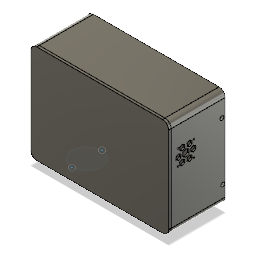
mouse_mock_MRI_box (Autodesk Fusion 360 design; units mm, degrees)
Autodesk Fusion 360 part; units mm, degrees
sketch "Sketch1" plane through (0, 0, 0) normal (0, 0, 1) x (1, 0, 0)
  line L0 (-140, 100) -> (140, 100)
  line L1 (140, 100) -> (140, -100)
  line L2 (140, -100) -> (-140, -100)
  line L3 (-140, -100) -> (-140, 100)
  line L4 (137, -97) -> (-137, -97)
  line L5 (-137, -97) -> (-137, 97)
  line L6 (-137, 97) -> (137, 97)
  line L7 (137, 97) -> (137, -97)
  dimension "d1" = 140
  dimension "d2" = 280
  dimension "d3" = 100
  dimension "d4" = 200
  dimension "d5" = 3
  constraint horizontal L0
  constraint vertical L1
  constraint horizontal L2
  constraint vertical L3
  measures "d1" distance of origin L3
  measures "d2" distance of L0.start L0.end
  measures "d3" distance of origin L0
  measures "d4" distance of L0.start L2.end
extrude "Extrude1" add sketch "Sketch1" along normal blind 10 contours L4 L5 L6 L7 makes body 1
extrude "Extrude2" add sketch "Sketch1" along normal blind 110 bodies 1
sketch "Sketch2" plane through (0, 0, 10) normal (0, 0, 1) x (1, 0, 0)
  line L0 (137, 97) -> (-137, 97)
  line L1 (-137, 97) -> (-137, -97)
  line L2 (-137, -97) -> (137, -97)
  line L3 (137, -97) -> (137, 97)
  line L4 (-30.5, 80) -> (-55.5, 80)
  line L5 (-55.5, 80) -> (-55.5, 10)
  line L6 (-55.5, 10) -> (-30.5, 10)
  line L7 (-30.5, 10) -> (-30.5, 80)
  line L8 (30.5, 80) -> (55.5, 80)
  line L9 (55.5, 80) -> (55.5, 10)
  line L10 (55.5, 10) -> (30.5, 10)
  line L11 (30.5, 10) -> (30.5, 80)
  line L12 (-9.5, -65) -> (9.5, -65)
  line L13 (9.5, -65) -> (9.5, -75.5)
  line L14 (9.5, -75.5) -> (-9.5, -75.5)
  line L15 (-9.5, -75.5) -> (-9.5, -65)
  circle A0 centre (-12.5, -70.25) radius 1.5
  circle A1 centre (12.5, -70.25) radius 1.5
  line L16 (-76.5, -65) -> (-95.5, -65)
  line L17 (-95.5, -65) -> (-95.5, -75.5)
  line L18 (-95.5, -75.5) -> (-76.5, -75.5)
  line L19 (-76.5, -75.5) -> (-76.5, -65)
  circle A2 centre (-73.5, -70.25) radius 1.5
  circle A3 centre (-98.5, -70.25) radius 1.5
  line L20 (0, 0) -> (0, -11.4681)
  circle A4 centre (98.5, -70.25) radius 1.5
  line L21 (95.5, -65) -> (95.5, -75.5)
  line L22 (95.5, -75.5) -> (76.5, -75.5)
  line L23 (76.5, -65) -> (95.5, -65)
  line L24 (76.5, -75.5) -> (76.5, -65)
  circle A5 centre (73.5, -70.25) radius 1.5
  line L25 (-116.5, 80) -> (-126.5, 80)
  line L26 (-126.5, 80) -> (-126.5, 10)
  line L27 (-126.5, 10) -> (-116.5, 10)
  line L28 (-116.5, 10) -> (-116.5, 80)
  line L29 (126.5, 80) -> (126.5, 10)
  line L30 (116.5, 80) -> (126.5, 80)
  line L31 (116.5, 10) -> (116.5, 80)
  line L32 (126.5, 10) -> (116.5, 10)
  line L33 (137, -97) -> (-137, -97)
  line L34 (-137, -97) -> (-137, -82.25)
  line L35 (-137, -82.25) -> (137, -82.25)
  line L36 (137, -82.25) -> (137, -97)
  line L37 (-116.5, -82.25) -> (-126.5, -82.25)
  line L38 (-126.5, -82.25) -> (-126.5, -72.25)
  line L39 (-126.5, -72.25) -> (-116.5, -72.25)
  line L40 (-116.5, -72.25) -> (-116.5, -82.25)
  line L41 (126.5, -82.25) -> (126.5, -72.25)
  line L42 (126.5, -72.25) -> (116.5, -72.25)
  line L43 (116.5, -72.25) -> (116.5, -82.25)
  line L44 (-30.5, -82.25) -> (-55.5, -82.25)
  line L45 (-55.5, -82.25) -> (-55.5, -72.25)
  line L46 (-55.5, -72.25) -> (-30.5, -72.25)
  line L47 (-30.5, -72.25) -> (-30.5, -82.25)
  line L48 (55.5, -82.25) -> (55.5, -72.25)
  line L49 (55.5, -72.25) -> (30.5, -72.25)
  line L50 (30.5, -72.25) -> (30.5, -82.25)
  dimension "d10" = 70
  dimension "d11" = 25
  dimension "d12" = 70
  dimension "d13" = 25
  dimension "d14" = 30.5
  dimension "d15" = 30.5
  dimension "d16" = 19
  dimension "d17" = 10.5
  dimension "d18" = 9.5
  dimension "d19" = 65
  dimension "d20" = 3
  dimension "d21" = 3
  dimension "d22" = 25
  dimension "d23" = 12.5
  dimension "d24" = 5.25
  dimension "d25" = 5.25
  dimension "d26" = 19
  dimension "d27" = 10.5
  dimension "d28" = 80
  dimension "d29" = 65
  dimension "d30" = 21
  dimension "d31" = 3
  dimension "d32" = 3
  dimension "d33" = 5.25
  dimension "d34" = 5.25
  dimension "d35" = 25
  dimension "d36" = 3
  dimension "d46" = 70
  dimension "d47" = 61
  dimension "d48" = 10
  dimension "d85" = 80
  dimension "d86" = 80
  dimension "d87" = 12
  dimension "d93" = 10
  dimension "d94" = 10
  constraint horizontal L4
  constraint vertical L5
  constraint horizontal L6
  constraint vertical L7
  constraint horizontal L8
  constraint vertical L9
  constraint horizontal L10
  constraint vertical L11
  constraint horizontal L12
  constraint vertical L13
  constraint horizontal L14
  constraint vertical L15
  constraint horizontal L16
  constraint vertical L17
  constraint horizontal L18
  constraint vertical L19
  constraint coincident L20.start origin
  constraint vertical L20
  constraint symmetric L16.start L20 L23.start
  constraint symmetric L16.end L20 L21.start
  constraint symmetric L17.end L20 L21.end
  constraint symmetric L18.end L20 L22.end
  constraint symmetric A2 L20 A5
  constraint symmetric A3 L20 A4
  constraint horizontal L25
  constraint vertical L26
  constraint horizontal L27
  constraint vertical L28
  constraint symmetric L20 L25.start L30.start
  constraint symmetric L20 L25.end L29.start
  constraint symmetric L20 L26.end L29.end
  constraint symmetric L20 L27.end L31.start
  constraint horizontal L33
  constraint vertical L34
  constraint horizontal L35
  constraint vertical L36
  constraint coincident L2 L3.start
  constraint coincident L1 L2.start
  constraint coincident L2.end L36
  constraint horizontal L37
  constraint vertical L38
  constraint horizontal L39
  constraint vertical L40
  constraint coincident L35 L37.start
  constraint symmetric L20 L37.start L43.end
  constraint symmetric L20 L37.end L41.start
  constraint symmetric L20 L38.end L41.end
  constraint symmetric L20 L39.end L42.end
  constraint horizontal L44
  constraint vertical L45
  constraint horizontal L46
  constraint vertical L47
  constraint coincident L35 L44.start
  constraint symmetric L20 L44.start L50.end
  constraint symmetric L20 L44.end L48.start
  constraint symmetric L20 L45.end L48.end
  constraint symmetric L20 L46.end L49.end
  measures "d10" distance of L4.start L6.end
  measures "d11" distance of L4.start L4.end
  measures "d12" distance of L8.start L10.end
  measures "d13" distance of L8.start L8.end
  measures "d14" distance of L20.start L7
  measures "d15" distance of L20.start L11
  measures "d16" distance of L12.start L12.end
  measures "d17" distance of L12.start L14.end
  measures "d18" distance of L20.start L15
  measures "d19" distance of L20.start L12
  measures "d20" diameter of A0
  measures "d21" diameter of A1
  measures "d22" distance of A0.centre A1.centre
  measures "d23" horizontal distance of L20.start A0.centre
  measures "d24" distance of L12 A0.centre
  measures "d25" distance of L12 A1.centre
  measures "d26" distance of L16.start L16.end
  measures "d27" distance of L16.start L18.end
  measures "d28" distance of L20.start L4
  measures "d29" distance of L20.start L16
  measures "d30" distance of L5 L19
  measures "d31" diameter of A2
  measures "d32" diameter of A3
  measures "d33" distance of L16 A2.centre
  measures "d34" distance of L16 A3.centre
  measures "d35" distance of A2.centre A3.centre
  measures "d36" distance of L17 A3.centre
  measures "d46" distance of L25.start L27.end
  measures "d47" distance of L5 L28
  measures "d48" distance of L25.start L25.end
  measures "d85" distance of L20.start L8
  measures "d86" distance of L20.start L25
  measures "d87" distance of A2.centre L35
  measures "d93" distance of L37.start L39.end
  measures "d94" distance of L44.start L46.end
extrude "Extrude3" add sketch "Sketch2" along normal blind 20 contours L4 L5 L6 L7 | L8 L9 L10 L11 | L25 L26 L27 L28 | L29 L30 L31 L32 bodies 1
extrude "Extrude4" cut sketch "Sketch2" against normal blind 9 contours L12 L13 L14 L15 | A0 | A1 | L16 L17 L18 L19 | A2 | A3 | A4 | L21 L22 L23 L24 | A5 bodies 1
sketch "Sketch3" plane through (140, 0, 0) normal (1, 0, 0) x (0, 0, -1)
  line L0 (0, -100) -> (0, 100)
  line L1 (0, 100) -> (-110, 100)
  line L2 (-110, 100) -> (-110, -100)
  line L3 (-110, -100) -> (0, -100)
  circle A0 centre (-5, -63) radius 4
  line L4 (0, 100) -> (0, -100)
  circle A1 centre (-80, 30) radius 20
  circle A2 centre (-96, 46) radius 1.5
  circle A3 centre (-96, 14) radius 1.5
  line L5 (-80, 40) -> (-80, 16.2892)
  circle A4 centre (-64, 14) radius 1.5
  circle A5 centre (-64, 46) radius 1.5
  line L6 (-90, 32.8868) -> (-95, 35.7735)
  line L7 (-95, 35.7735) -> (-100, 32.8868)
  line L8 (-100, 32.8868) -> (-100, 27.1132)
  line L9 (-100, 27.1132) -> (-95, 24.2265)
  line L10 (-95, 24.2265) -> (-90, 27.1132)
  line L11 (-90, 27.1132) -> (-90, 32.8868)
  line L12 (-87.5, 22.7831) -> (-92.5, 19.8964)
  line L13 (-92.5, 19.8964) -> (-92.5, 14.1229)
  line L14 (-92.5, 14.1229) -> (-87.5, 11.2361)
  line L15 (-87.5, 11.2361) -> (-82.5, 14.1229)
  line L16 (-82.5, 19.8964) -> (-87.5, 22.7831)
  line L17 (-82.5, 14.1229) -> (-82.5, 19.8964)
  line L18 (-77.5, 19.8964) -> (-77.5, 14.1229)
  line L19 (-77.5, 14.1229) -> (-72.5, 11.2361)
  line L20 (-72.5, 11.2361) -> (-67.5, 14.1229)
  line L21 (-67.5, 14.1229) -> (-67.5, 19.8964)
  line L22 (-72.5, 22.7831) -> (-77.5, 19.8964)
  line L23 (-67.5, 19.8964) -> (-72.5, 22.7831)
  line L24 (-70, 27.1132) -> (-65, 24.2265)
  line L25 (-65, 24.2265) -> (-60, 27.1132)
  line L26 (-60, 27.1132) -> (-60, 32.8868)
  line L27 (-60, 32.8868) -> (-65, 35.7735)
  line L28 (-70, 32.8868) -> (-70, 27.1132)
  line L29 (-65, 35.7735) -> (-70, 32.8868)
  line L30 (-72.5, 37.2169) -> (-67.5, 40.1036)
  line L31 (-67.5, 40.1036) -> (-67.5, 45.8771)
  line L32 (-67.5, 45.8771) -> (-72.5, 48.7639)
  line L33 (-72.5, 48.7639) -> (-77.5, 45.8771)
  line L34 (-77.5, 40.1036) -> (-72.5, 37.2169)
  line L35 (-77.5, 45.8771) -> (-77.5, 40.1036)
  line L36 (-82.5, 40.1036) -> (-82.5, 45.8771)
  line L37 (-82.5, 45.8771) -> (-87.5, 48.7639)
  line L38 (-87.5, 48.7639) -> (-92.5, 45.8771)
  line L39 (-92.5, 45.8771) -> (-92.5, 40.1036)
  line L40 (-87.5, 37.2169) -> (-82.5, 40.1036)
  line L41 (-92.5, 40.1036) -> (-87.5, 37.2169)
  line L42 (-73.5687, 33.7131) -> (-80, 37.4262)
  line L43 (-80, 37.4262) -> (-86.4313, 33.7131)
  line L44 (-86.4313, 33.7131) -> (-86.4313, 26.2869)
  line L45 (-86.4313, 26.2869) -> (-80, 22.5738)
  line L46 (-80, 22.5738) -> (-73.5687, 26.2869)
  line L47 (-73.5687, 26.2869) -> (-73.5687, 33.7131)
  point P0 (-64, 46)
  point P1 (-64, 14)
  point P2 (-95, 30)
  point P3 (-80, 30)
  dimension "d41" = 8
  dimension "d42" = 63
  dimension "d43" = 5
  dimension "d49" = 40
  dimension "d50" = 30
  dimension "d51" = 80
  dimension "d52" = 3
  dimension "d53" = 16
  dimension "d54" = 16
  dimension "d55" = 3
  dimension "d56" = 16
  dimension "d57" = 16
  dimension "d127" = 360
  constraint vertical L5
  constraint symmetric A2.centre L5 P0
  constraint symmetric A3.centre L5 P1
  constraint symmetric A2 L5 A5
  constraint symmetric A3 L5 A4
  constraint coincident P3 A1.centre
  measures "d41" diameter of A0
  measures "d42" vertical distance of origin A0.centre
  measures "d43" distance of A0.centre L4
  measures "d49" diameter of A1
  measures "d50" vertical distance of origin P3
  measures "d51" horizontal distance of P3 origin
  measures "d52" diameter of A2
  measures "d53" vertical distance of P3 A2.centre
  measures "d54" horizontal distance of P3 A2.centre
  measures "d55" diameter of A3
  measures "d56" vertical distance of P3 A3.centre
  measures "d57" horizontal distance of P3 A3.centre
extrude "Extrude5" cut sketch "Sketch3" against normal blind 335 contours A1 L24 L25 L27 L28 L29 | A1 L30 L31 L33 L34 L35 | A1 L18 L19 L21 L22 L23 | A1 L36 L37 L39 L40 L41 | A1 L12 L13 L15 L16 L17 | A1 L6 L7 L9 L10 L11 | L5 L42 L46 L47 | L5 L43 L44 L45 bodies 1
extrude "Extrude6" cut sketch "Sketch3" against normal blind 9 contours A2 | A3 | A4 | A5 bodies 1
sketch "Sketch4" plane through (0, 0, 10) normal (0, 0, 1) x (1, 0, 0)
  circle A0 centre (73.5, -70.25) radius 1.5
  circle A1 centre (-98.5, -70.25) radius 1.5
  circle A2 centre (-73.5, -70.25) radius 1.5
  circle A3 centre (12.5, -70.25) radius 1.5
  line L0 (95.5, -65) -> (95.5, -75.5)
  line L1 (95.5, -75.5) -> (76.5, -75.5)
  line L2 (76.5, -75.5) -> (76.5, -65)
  line L3 (76.5, -65) -> (95.5, -65)
  circle A4 centre (-12.5, -70.25) radius 1.5
  line L4 (-95.5, -65) -> (-76.5, -65)
  line L5 (-76.5, -65) -> (-76.5, -75.5)
  line L6 (-76.5, -75.5) -> (-95.5, -75.5)
  line L7 (-95.5, -75.5) -> (-95.5, -65)
  line L8 (9.5, -65) -> (9.5, -75.5)
  line L9 (9.5, -75.5) -> (-9.5, -75.5)
  line L10 (-9.5, -75.5) -> (-9.5, -65)
  line L11 (-9.5, -65) -> (9.5, -65)
  circle A5 centre (98.5, -70.25) radius 1.5
  line L12 (126.5, 10) -> (116.5, 10)
  line L13 (116.5, 10) -> (116.5, 80)
  line L14 (116.5, 80) -> (126.5, 80)
  line L15 (126.5, 80) -> (126.5, 10)
  line L16 (-30.5, 10) -> (-55.5, 10)
  line L17 (-55.5, 10) -> (-55.5, 80)
  line L18 (-55.5, 80) -> (-30.5, 80)
  line L19 (-30.5, 80) -> (-30.5, 10)
  line L20 (-116.5, 10) -> (-126.5, 10)
  line L21 (-126.5, 10) -> (-126.5, 80)
  line L22 (-126.5, 80) -> (-116.5, 80)
  line L23 (-116.5, 80) -> (-116.5, 10)
  line L24 (30.5, 10) -> (30.5, 80)
  line L25 (30.5, 80) -> (55.5, 80)
  line L26 (55.5, 80) -> (55.5, 10)
  line L27 (55.5, 10) -> (30.5, 10)
  line L28 (137, 97) -> (-137, 97)
  line L29 (-137, 97) -> (-137, -97)
  line L30 (-137, -97) -> (137, -97)
  line L31 (137, -97) -> (137, 97)
  line L32 (137, 50) -> (125, 50)
  line L33 (125, 50) -> (125, 62)
  line L34 (125, 62) -> (137, 62)
  line L35 (137, 62) -> (137, 50)
  line L36 (135, 52) -> (127, 52)
  line L37 (127, 52) -> (127, 60)
  line L38 (127, 60) -> (135, 60)
  line L39 (135, 60) -> (135, 52)
  dimension "d62" = 12
  dimension "d63" = 12
  dimension "d75" = 2
  dimension "d76" = 50
  constraint horizontal L32
  constraint vertical L33
  constraint horizontal L34
  constraint vertical L35
  constraint coincident L31 L32.start
  measures "d62" distance of L32.start L32.end
  measures "d63" distance of L32.start L34.end
  measures "d76" distance of origin L32
extrude "Extrude7" add sketch "Sketch4" along normal blind 90 contours L15 L32 L33 L34 | L15 L31 L32 L34 L35 bodies 1
extrude "Extrude8" cut 1 faces at (129.6667, 54.6667, 10) along direction (0, 0, -1) blind 9 on bodies 1 bodies 1
sketch "Sketch5" plane through (140, 0, 0) normal (1, 0, 0) x (0, 0, -1)
  circle A0 centre (-96, 14) radius 1.5
  circle A1 centre (-64, 46) radius 1.5
  circle A2 centre (-96, 46) radius 1.5
  circle A3 centre (-64, 14) radius 1.5
  line L0 (0, -100) -> (0, 100)
  line L1 (0, 100) -> (-110, 100)
  line L2 (-110, 100) -> (-110, -100)
  line L3 (-110, -100) -> (0, -100)
  circle A4 centre (-7, 54.7292) radius 4
  line L4 (-72.5, 37.2169) -> (-77.5, 40.1036)
  line L5 (-77.5, 40.1036) -> (-77.5, 45.8771)
  line L6 (-77.5, 45.8771) -> (-72.7292, 48.6316)
  arc A5 (-67.5, 45.6125) -> (-72.7292, 48.6316) centre (-80, 30) ccw
  line L7 (-67.5, 45.6125) -> (-67.5, 40.1036)
  line L8 (-67.5, 40.1036) -> (-72.5, 37.2169)
  line L9 (-95, 35.7735) -> (-90, 32.8868)
  line L10 (-90, 32.8868) -> (-90, 27.1132)
  line L11 (-90, 27.1132) -> (-95, 24.2265)
  line L12 (-95, 24.2265) -> (-99.7708, 26.9809)
  arc A6 (-99.7708, 33.0191) -> (-99.7708, 26.9809) centre (-80, 30) ccw
  line L13 (-99.7708, 33.0191) -> (-95, 35.7735)
  line L14 (-87.5, 22.7831) -> (-82.5, 19.8964)
  line L15 (-82.5, 19.8964) -> (-82.5, 14.1229)
  line L16 (-82.5, 14.1229) -> (-87.2708, 11.3684)
  arc A7 (-92.5, 14.3875) -> (-87.2708, 11.3684) centre (-80, 30) ccw
  line L17 (-92.5, 14.3875) -> (-92.5, 19.8964)
  line L18 (-92.5, 19.8964) -> (-87.5, 22.7831)
  line L19 (-77.5, 19.8964) -> (-72.5, 22.7831)
  line L20 (-72.5, 22.7831) -> (-67.5, 19.8964)
  line L21 (-67.5, 19.8964) -> (-67.5, 14.3875)
  arc A8 (-72.7292, 11.3684) -> (-67.5, 14.3875) centre (-80, 30) ccw
  line L22 (-72.7292, 11.3684) -> (-77.5, 14.1229)
  line L23 (-77.5, 14.1229) -> (-77.5, 19.8964)
  line L24 (-82.5, 40.1036) -> (-87.5, 37.2169)
  line L25 (-87.5, 37.2169) -> (-92.5, 40.1036)
  line L26 (-92.5, 40.1036) -> (-92.5, 45.6125)
  arc A9 (-87.2708, 48.6316) -> (-92.5, 45.6125) centre (-80, 30) ccw
  line L27 (-87.2708, 48.6316) -> (-82.5, 45.8771)
  line L28 (-82.5, 45.8771) -> (-82.5, 40.1036)
  line L29 (-70, 27.1132) -> (-70, 32.8868)
  line L30 (-70, 32.8868) -> (-65, 35.7735)
  line L31 (-65, 35.7735) -> (-60.2292, 33.0191)
  arc A10 (-60.2292, 26.9809) -> (-60.2292, 33.0191) centre (-80, 30) ccw
  line L32 (-60.2292, 26.9809) -> (-65, 24.2265)
  line L33 (-65, 24.2265) -> (-70, 27.1132)
  line L34 (-80, 37.4262) -> (-73.5687, 33.7131)
  line L35 (-73.5687, 33.7131) -> (-73.5687, 26.2869)
  line L36 (-73.5687, 26.2869) -> (-80, 22.5738)
  line L37 (-80, 22.5738) -> (-86.4313, 26.2869)
  line L38 (-86.4313, 26.2869) -> (-86.4313, 33.7131)
  line L39 (-86.4313, 33.7131) -> (-80, 37.4262)
  dimension "d69" = 8
  dimension "d70" = 7
  measures "d69" diameter of A4
  measures "d70" horizontal distance of origin A4.centre
extrude "Extrude9" cut sketch "Sketch5" against normal blind 10 contours A4 bodies 1
sketch "Sketch6" plane through (0, 0, 100) normal (0, 0, 1) x (1, 0, 0)
  line L0 (127, 60) -> (135, 60)
  line L1 (135, 60) -> (135, 52)
  line L2 (135, 52) -> (127, 52)
  line L3 (127, 52) -> (127, 60)
  line L4 (137, 62) -> (125, 62)
  line L5 (125, 62) -> (125, 50)
  line L6 (125, 50) -> (137, 50)
  line L7 (137, 50) -> (137, 62)
  line L8 (125, 62) -> (125, 50)
  line L9 (137, 62) -> (125, 62)
  line L10 (125, 50) -> (137, 50)
  line L11 (137, 62) -> (137, 50)
extrude "Extrude10" add sketch "Sketch6" along normal blind 2 contours L0 L1 L2 L3 | L4 L5 L6 L7 L8 L9 L10 L11 bodies 1
sketch "Sketch7" plane through (0, 50, 0) normal (0, -1, 0) x (1, 0, 0)
  line L0 (125, 30) -> (126.5, 30)
  line L1 (126.5, 30) -> (126.5, 10)
  line L2 (126.5, 10) -> (137, 10)
  line L3 (137, 10) -> (137, 102)
  line L4 (137, 102) -> (125, 102)
  line L5 (125, 102) -> (125, 30)
  line L6 (130, 95) -> (135, 95)
  line L7 (135, 95) -> (135, 65)
  line L8 (135, 65) -> (130, 65)
  line L9 (130, 65) -> (130, 95)
  constraint horizontal L6
  constraint vertical L7
  constraint horizontal L8
  constraint vertical L9
extrude "Extrude11" cut sketch "Sketch7" against normal blind 5 contours L6 L7 L8 L9 bodies 1
fillet "Fillet1" radius 10 4 edges at (137, 97, 60) (137, -97, 60) (-137, 97, 60) (-137, -97, 60) on bodies 1
extrude "Extrude12" cut sketch "Sketch3" against normal blind 235 contours A0 bodies 1
extrude "Extrude13" add sketch "Sketch2" along normal blind 30 contours L1 L2 L3 L33 L34 L35 L36 L37 L44 | L35 L41 L42 L43 | L35 L37 L38 L39 L40 | L35 L48 L49 L50 | L35 L44 L45 L46 L47 bodies 1
fillet "Fillet3" radius 12.5 4 edges at (140, -100, 55) (-140, -100, 55) (140, 100, 55) (-140, 100, 55) on bodies 1
chamfer "Chamfer1" distance 5 distance2 20 5 edges at (-131.75, -82.25, 40) (131.75, -82.25, 40) (86, -82.25, 40) (0, -82.25, 40) (-86, -82.25, 40) measured on face at (-10.1667, -92.0833, 40) measured on face at (-10.1667, -92.0833, 40) measured on face at (-10.1667, -92.0833, 40) measured on face at (-10.1667, -92.0833, 40) measured on face at (-10.1667, -92.0833, 40) on bodies 1
chamfer "Chamfer2" distance 10 distance2 25 4 edges at (121.5, -72.25, 40) (43, -72.25, 40) (-43, -72.25, 40) (-121.5, -72.25, 40) measured on face at (-47.1667, -77.25, 40) measured on face at (-47.1667, -77.25, 40) measured on face at (-47.1667, -77.25, 40) measured on face at (-47.1667, -77.25, 40) on bodies 1
chamfer "Chamfer3" distance 3 distance2 15 14 edges at (55.5, 45, 30) (43, 10, 30) (30.5, 45, 30) (43, 80, 30) (-43, 10, 30) (-30.5, 45, 30) (-55.5, 45, 30) (-43, 80, 30) (116.5, 45, 30) (121.5, 10, 30) (121.5, 80, 30) (-116.5, 45, 30) (-121.5, 10, 30) (-121.5, 80, 30) measured on face at (38.8333, 56.6667, 30) measured on face at (38.8333, 56.6667, 30) measured on face at (38.8333, 56.6667, 30) measured on face at (38.8333, 56.6667, 30) measured on face at (-47.1667, 56.6667, 30) measured on face at (-47.1667, 56.6667, 30) measured on face at (-47.1667, 56.6667, 30) measured on face at (-47.1667, 56.6667, 30) measured on face at (122.6667, 23.3333, 30) measured on face at (122.6667, 23.3333, 30) measured on face at (122.6667, 23.3333, 30) measured on face at (-123.1667, 56.6667, 30) measured on face at (-123.1667, 56.6667, 30) measured on face at (-123.1667, 56.6667, 30) on bodies 1
sketch "Sketch8" plane through (0, 0, 110) normal (0, 0, 1) x (1, 0, 0)
  arc A0 (-127.5, 100) -> (-140, 87.5) centre (-127.5, 87.5) ccw
  line L0 (-140, 87.5) -> (-140, -87.5)
  arc A1 (-140, -87.5) -> (-127.5, -100) centre (-127.5, -87.5) ccw
  line L1 (-127.5, -100) -> (127.5, -100)
  arc A2 (127.5, -100) -> (140, -87.5) centre (127.5, -87.5) ccw
  line L2 (140, -87.5) -> (140, 87.5)
  arc A3 (140, 87.5) -> (127.5, 100) centre (127.5, 87.5) ccw
  line L3 (127.5, 100) -> (-127.5, 100)
  line L4 (-127, 97) -> (127, 97)
  arc A4 (137, 87) -> (127, 97) centre (127, 87) ccw
  line L5 (137, 87) -> (137, -87)
  arc A5 (127, -97) -> (137, -87) centre (127, -87) ccw
  line L6 (127, -97) -> (-127, -97)
  arc A6 (-137, -87) -> (-127, -97) centre (-127, -87) ccw
  line L7 (-137, -87) -> (-137, 87)
  arc A7 (-127, 97) -> (-137, 87) centre (-127, 87) ccw
  arc A8 (138, 87) -> (127, 98) centre (127, 87) ccw
  line L8 (-127, 98) -> (127, 98)
  arc A9 (-127, 98) -> (-138, 87) centre (-127, 87) ccw
  line L9 (-138, -87) -> (-138, 87)
  arc A10 (-138, -87) -> (-127, -98) centre (-127, -87) ccw
  line L10 (127, -98) -> (-127, -98)
  arc A11 (127, -98) -> (138, -87) centre (127, -87) ccw
  line L11 (138, 87) -> (138, -87)
  dimension "d99" = -1
extrude "Extrude14" add sketch "Sketch8" along normal blind 5 separate body contours A0 L0 A1 L1 A2 L2 A3 L3 | L4 A4 L5 A5 L6 A6 L7 A7 | A8 L8 A9 L9 A10 L10 A11 L11 makes body 2
extrude "Extrude15" add sketch "Sketch8" against normal blind 3 contours L4 A4 L5 A5 L6 A6 L7 A7 bodies 2
sketch "Sketch9" plane through (0, -100, 0) normal (0, -1, 0) x (1, 0, 0)
  line L0 (-127.5, 110) -> (-127.5, 0)
  line L1 (-127.5, 0) -> (127.5, 0)
  line L2 (127.5, 0) -> (127.5, 110)
  line L3 (127.5, 110) -> (-127.5, 110)
  circle A0 centre (0, 55) radius 30.5
  circle A1 centre (-86, 55) radius 30.5
  circle A2 centre (86, 55) radius 30.5
  circle A3 centre (-86, 93) radius 2
  circle A4 centre (-86, 93) radius 5
  circle A5 centre (0, 93) radius 5
  circle A6 centre (0, 93) radius 2
  circle A7 centre (86, 93) radius 5
  circle A8 centre (86, 93) radius 2
  circle A9 centre (-86, 17) radius 5
  circle A10 centre (-86, 17) radius 2
  circle A11 centre (0, 17) radius 5
  circle A12 centre (0, 17) radius 2
  circle A13 centre (86, 17) radius 5
  circle A14 centre (86, 17) radius 2
  dimension "d106" = 61
  dimension "d107" = 55
  dimension "d108" = 61
  dimension "d109" = 86
  dimension "d110" = 61
  dimension "d111" = 86
  dimension "d112" = 4
  dimension "d113" = 38
  dimension "d114" = 10
  dimension "d117" = 172
  dimension "d118" = -76
  constraint concentric A3 A4
  measures "d106" diameter of A0
  measures "d107" distance of origin A0.centre
  measures "d108" diameter of A1
  measures "d109" distance of A0.centre A1.centre
  measures "d110" diameter of A2
  measures "d111" distance of A0.centre A2.centre
  measures "d112" diameter of A3
  measures "d113" distance of A1.centre A3.centre
  measures "d114" diameter of A4
extrude "Extrude16" add sketch "Sketch9" against normal blind 7 contours A4 | A5 | A7 | A9 | A11 | A13 bodies 1
extrude "Extrude17" cut sketch "Sketch9" against normal blind 20 contours A0 | A1 | A2 bodies 1
extrude "Extrude18" cut sketch "Sketch9" against normal blind 6 contours A3 | A6 | A8 | A10 | A12 | A14 bodies 1
chamfer "Chamfer4" distance 4 angle 45 3 edges at (-90.6616, -97, 91.1919) (-4.6616, -97, 91.1919) (81.3384, -97, 91.1919) on bodies 1
sketch "Sketch10" plane through (0, -100, 0) normal (0, -1, 0) x (1, 0, 0)
  circle A0 centre (-86, 55) radius 30.5
  circle A1 centre (-86, 93) radius 5
  circle A2 centre (-86, 93) radius 2
  circle A3 centre (-86, 17) radius 5
  circle A4 centre (-86, 17) radius 2
  circle A5 centre (-86, 55) radius 32.5
  circle A6 centre (-86, 93) radius 7
  circle A7 centre (-86, 17) radius 7
  circle A8 centre (-86, 93) radius 1.6
  circle A9 centre (-86, 17) radius 1.6
  dimension "d128" = 65
  dimension "d129" = 14
  dimension "d130" = 14
  dimension "d187" = 3.2
  dimension "d188" = 3.2
  constraint concentric A0 A5
  constraint concentric A2 A6
  constraint concentric A3 A7
  constraint concentric A1 A8
  constraint concentric A4 A9
  measures "d128" diameter of A5
  measures "d129" diameter of A6
  measures "d130" diameter of A7
  measures "d187" diameter of A8
  measures "d188" diameter of A9
extrude "Extrude19" add sketch "Sketch10" sketch "Sketch9" along normal blind 15 separate body contours A1 | A2 | A3 | A4 | A5 A6 A7 | A5 A6 | A5 A6 | A5 A7 | A5 A7 of sketch 2 contours A1 | A4 makes body 3
sketch "Sketch11" plane through (0, -100, 0) normal (0, 1, 0) x (-1, 0, 0)
  arc A0 (82.0031, 22.7467) -> (89.9969, 22.7467) centre (86, 17) ccw
  arc A1 (89.9969, 22.7467) -> (89.9969, 87.2533) centre (86, 55) ccw
  arc A2 (89.9969, 87.2533) -> (82.0031, 87.2533) centre (86, 93) ccw
  arc A3 (82.0031, 87.2533) -> (82.0031, 22.7467) centre (86, 55) ccw
  circle A4 centre (86, 55) radius 30.5
  circle A5 centre (86, 55) radius 29
  line L0 (89.5, 76.5) -> (82.5, 76.5)
  line L1 (82.5, 76.5) -> (82.5, 82.5)
  line L2 (82.5, 82.5) -> (89.5, 82.5)
  line L3 (89.5, 82.5) -> (89.5, 76.5)
  circle A6 centre (86, 55) radius 13.5
  circle A7 centre (86, 17) radius 1.6
  circle A8 centre (86, 93) radius 1.6
  dimension "d133" = 61
  dimension "d134" = 58
  dimension "d135" = 7
  dimension "d136" = 6
  dimension "d137" = 3.5
  dimension "d138" = 27.5
  dimension "d153" = 27
  constraint concentric A1 A4
  constraint concentric A1 A5
  constraint horizontal L0
  constraint vertical L1
  constraint horizontal L2
  constraint vertical L3
  constraint concentric A4 A6
  measures "d133" diameter of A4
  measures "d134" diameter of A5
  measures "d135" distance of L0.start L0.end
  measures "d136" distance of L0.start L2.end
  measures "d137" distance of A1.centre L3
  measures "d138" distance of A1.centre L2
  measures "d153" diameter of A6
extrude "Extrude20" cut sketch "Sketch11" against normal blind 13 contours A5 | L0 L1 L2 L3 | A6 bodies 3
extrude "Extrude21" cut sketch "Sketch11" against normal blind 6 contours A4 bodies 3
fillet "Fillet4" radius 3.5 4 edges at (-82.0031, -107.5, 87.2533) (-82.0031, -107.5, 22.7467) (-89.9969, -107.5, 22.7467) (-89.9969, -107.5, 87.2533) on bodies 3
sketch "Sketch12" plane through (0, -115, 0) normal (0, -1, 0) x (1, 0, 0)
  arc A0 (-92.6233, 19.2654) -> (-79.3767, 19.2654) centre (-86, 17) ccw
  arc A1 (-77.0309, 23.7621) -> (-79.3767, 19.2654) centre (-76.065, 20.398) ccw
  arc A2 (-77.0309, 23.7621) -> (-77.0309, 86.2379) centre (-86, 55) ccw
  arc A3 (-79.3767, 90.7346) -> (-77.0309, 86.2379) centre (-76.065, 89.602) ccw
  arc A4 (-79.3767, 90.7346) -> (-92.6233, 90.7346) centre (-86, 93) ccw
  arc A5 (-94.9691, 86.2379) -> (-92.6233, 90.7346) centre (-95.935, 89.602) ccw
  arc A6 (-94.9691, 86.2379) -> (-94.9691, 23.7621) centre (-86, 55) ccw
  arc A7 (-92.6233, 19.2654) -> (-94.9691, 23.7621) centre (-95.935, 20.398) ccw
  circle A8 centre (-86, 93) radius 2.9
  circle A9 centre (-86, 17) radius 2.9
  circle A10 centre (-86, 17) radius 1.6
  circle A11 centre (-86, 93) radius 1.6
  dimension "d147" = 5.8
  dimension "d148" = 5.8
  measures "d147" diameter of A8
  measures "d148" diameter of A9
extrude "Extrude23" cut sketch "Sketch12" against normal blind 5 contours A8 | A9 | A10 | A11 bodies 3
chamfer "Chamfer5" distance 1 distance2 12 8 edges at (-118.5, -115, 55) (-92.8318, -115, 22.0168) (-86, -115, 10) (-79.1682, -115, 22.0168) (-53.5, -115, 55) (-79.1682, -115, 87.9832) (-86, -115, 100) (-92.8318, -115, 87.9832) measured on face at (-88.6581, -115, 39.9725) measured on face at (-92.7011, -110, 21.7368) measured on face at (-88.6581, -115, 39.9725) measured on face at (-79.2327, -105, 21.8865) measured on face at (-88.6581, -115, 39.9725) measured on face at (-79.0983, -105, 87.8557) measured on face at (-88.6581, -115, 39.9725) measured on face at (-92.9867, -105, 87.7158) on bodies 3
extrude "Extrude24" cut sketch "Sketch11" against normal blind 40 contours A6 bodies 3
sketch "Sketch14" plane through (0, -113, 0) normal (0, 1, 0) x (-1, 0, 0)
  circle A0 centre (86, 55) radius 13.5
  circle A1 centre (86, 55) radius 29
  circle A2 centre (86, 55) radius 17
  dimension "d156" = 34
  constraint concentric A0 A2
  measures "d156" diameter of A2
extrude "Extrude25" add sketch "Sketch14" along normal blind 7 contours A2 bodies 3
sketch "Sketch15" plane through (0, -106, 0) normal (0, 1, 0) x (-1, 0, 0)
  circle A0 centre (86, 55) radius 29
  circle A1 centre (86, 55) radius 30.5
  circle A2 centre (85.8466, 24.5004) radius 1
  circle A3 centre (85.8466, 85.4996) radius 1
  dimension "d159" = 2
  dimension "d160" = 2
  constraint coincident A1 A2.centre
  constraint coincident A1 A3.centre
  measures "d159" diameter of A2
  measures "d160" diameter of A3
extrude "Extrude26" add sketch "Sketch15" along normal blind 3 contours A1 A3 | A1 A2 picked at (85.8236, 85.1659) picked at (85.8236, 24.8341) bodies 3
fillet "Fillet5" radius 3.5 2 edges at (-70.1504, -113, 61.1475) (-58.9625, -113, 65.4868) on bodies 3
sketch "Sketch17" plane through (0, -106, 0) normal (0, 1, 0) x (-1, 0, 0)
  circle A0 centre (86, 55) radius 13.5
  circle A1 centre (86, 55) radius 17
  circle A2 centre (86, 55) radius 15.75
  dimension "d169" = 31.5
  constraint concentric A0 A2
  measures "d169" diameter of A2
extrude "Extrude28" add sketch "Sketch17" along normal blind 10 contours A2 bodies 3
sketch "Sketch18" plane through (0, -115, 0) normal (0, -1, 0) x (1, 0, 0)
  circle A0 centre (-86, 55) radius 13.5
  circle A1 centre (-86, 17) radius 2.9
  circle A2 centre (-86, 93) radius 2.9
  arc A3 (-80.3229, 91.0583) -> (-91.6771, 91.0583) centre (-86, 93) ccw
  arc A4 (-94.6931, 85.2767) -> (-91.6771, 91.0583) centre (-95.935, 89.602) ccw
  arc A5 (-94.6931, 85.2767) -> (-94.6931, 24.7233) centre (-86, 55) ccw
  arc A6 (-91.6771, 18.9417) -> (-94.6931, 24.7233) centre (-95.935, 20.398) ccw
  arc A7 (-91.6771, 18.9417) -> (-80.3229, 18.9417) centre (-86, 17) ccw
  arc A8 (-77.3069, 24.7233) -> (-80.3229, 18.9417) centre (-76.065, 20.398) ccw
  arc A9 (-77.3069, 24.7233) -> (-77.3069, 85.2767) centre (-86, 55) ccw
  arc A10 (-80.3229, 91.0583) -> (-77.3069, 85.2767) centre (-76.065, 89.602) ccw
  line L0 (-90.5, 67) -> (-81.5, 67)
  line L1 (-81.5, 67) -> (-81.5, 67)
  line L2 (-85.5, 71) -> (-86.5, 71)
  line L3 (-90.5, 67) -> (-90.5, 67)
  arc A11 (-81.5, 67) -> (-85.5, 71) centre (-85.5, 67) ccw
  arc A12 (-86.5, 71) -> (-90.5, 67) centre (-86.5, 67) ccw
  dimension "d172" = 9
  dimension "d174" = 12
  dimension "d176" = 16
  dimension "d177" = 4
  constraint horizontal L0
  constraint horizontal L2
  constraint tangent L2 A11
  constraint tangent L2 A12
  constraint equal A11 A12
  measures "d172" distance of L0.start L0.end
  measures "d174" distance of A0.centre L0
  measures "d176" distance of A0.centre L2
  measures "d177" radius of A11
extrude "Extrude29" cut sketch "Sketch18" against normal blind 5 contours A0 L2 A11 A12 bodies 3
sketch "Sketch19" plane through (0, -110, 0) normal (0, -1, 0) x (1, 0, 0)
  arc A0 (-81.5715, 67.753) -> (-85.5, 71) centre (-85.5, 67) ccw
  line L0 (-85.5, 71) -> (-86.5, 71)
  arc A1 (-86.5, 71) -> (-90.4285, 67.753) centre (-86.5, 67) ccw
  arc A2 (-81.5715, 67.753) -> (-90.4285, 67.753) centre (-86, 55) ccw
  line L1 (-86, 55) -> (-86, 93) construction
  line L2 (-86, 68.5) -> (-86, 71)
  constraint coincident A2.centre L1.start
  constraint vertical L1
  constraint midpoint A2 L2.start
  constraint midpoint L0 L2.end
revolve "Revolve1" cut sketch "Sketch19" angle 360 about axis through (-86, -110, 55) along (0, 0, 1) contours L0 A1 A2 L2 bodies 3
sketch "Sketch20" plane through (0, -115, 0) normal (0, -1, 0) x (1, 0, 0)
  arc A0 (-81.5715, 67.753) -> (-85.5, 71) centre (-85.5, 67) ccw
  arc A1 (-90.4285, 67.753) -> (-81.5715, 67.753) centre (-86, 55) ccw
  arc A2 (-86.5, 71) -> (-90.4285, 67.753) centre (-86.5, 67) ccw
  line L0 (-86.5, 71) -> (-85.5, 71)
  circle A3 centre (-86, 17) radius 2.9
  circle A4 centre (-86, 93) radius 2.9
  arc A5 (-80.3229, 91.0583) -> (-91.6771, 91.0583) centre (-86, 93) ccw
  arc A6 (-94.6931, 85.2767) -> (-91.6771, 91.0583) centre (-95.935, 89.602) ccw
  arc A7 (-94.6931, 85.2767) -> (-94.6931, 24.7233) centre (-86, 55) ccw
  arc A8 (-91.6771, 18.9417) -> (-94.6931, 24.7233) centre (-95.935, 20.398) ccw
  arc A9 (-91.6771, 18.9417) -> (-80.3229, 18.9417) centre (-86, 17) ccw
  arc A10 (-77.3069, 24.7233) -> (-80.3229, 18.9417) centre (-76.065, 20.398) ccw
  arc A11 (-77.3069, 24.7233) -> (-77.3069, 85.2767) centre (-86, 55) ccw
  arc A12 (-80.3229, 91.0583) -> (-77.3069, 85.2767) centre (-76.065, 89.602) ccw
  line L1 (-99.3, 55.5) -> (-100.3, 55.5)
  line L2 (-100.3, 55.5) -> (-100.3, 54.5)
  line L3 (-100.3, 54.5) -> (-99.3, 54.5)
  line L4 (-99.3, 54.5) -> (-99.3, 55.5)
  line L5 (-72.7, 54.5) -> (-71.7, 54.5)
  line L6 (-71.7, 54.5) -> (-71.7, 55.5)
  line L7 (-71.7, 55.5) -> (-72.7, 55.5)
  line L8 (-72.7, 55.5) -> (-72.7, 54.5)
  circle A13 centre (-86, 55) radius 13.5
  circle A14 centre (-86, 55) radius 13.5
  circle A15 centre (-86, 55) radius 15.75
  dimension "d183" = 13.3
  dimension "d184" = 13.3
  constraint horizontal L1
  constraint vertical L2
  constraint horizontal L3
  constraint vertical L4
  constraint horizontal L5
  constraint vertical L6
  constraint horizontal L7
  constraint vertical L8
  measures "d183" distance of L8 A1.centre
  measures "d184" distance of L4 A1.centre
extrude "Extrude30" add sketch "Sketch20" against normal blind 19 contours A1 L5 L7 L8 A13 A14 | A1 L1 L3 L4 A13 A14 bodies 3
chamfer "Chamfer7" distance 0.1 distance2 19 2 edges at (-72.7, -115, 55) (-99.3, -115, 55) measured on face at (-86.3284, -115, 29.7962) measured on face at (-86.3284, -115, 29.7962) on bodies 3
